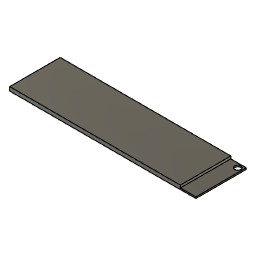
X-Axis Sensor Elevator (Autodesk Fusion 360 design; units mm, degrees)
Autodesk Fusion 360 part; units mm, degrees
box "BoxPrimitive1" add length 41.3548 width 139.7 height 3.175 placed x (0, -1, 0) y (1, 0, 0) z (0, 0, 1) at (0, 0, 0)
box "BoxPrimitive2" add length 41.275 width 29.6956 height 1.143 placed x (0, -1, 0) y (1, 0, 0) z (0, 0, 1) at (122.7007, -0.0274, 0)
hole "Hole1" at (148.831, -3.4125, 1.143) direction (0, 0, -1) diameter 5.08 depth 15.24 tip angle 180
